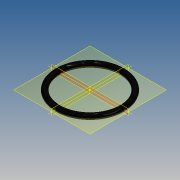
# Autodesk Inventor part: P030_OringCam
Saved by Autodesk Inventor 2021.3 (Build 253353000, 353)
## iProperties
Created: 2021-11-19
Part Number: P030_OringCam
Material: Générique
Document SubType Name: Modeling
Designer: gabri
Density: 1 g/cm^3
Appearance: Black
Author: gabri
Autodesk Inventor part; units mm, degrees
sketch "Sketch2" plane through (0, 0, 0) normal (0, 0, 1) x (1, 0, 0)
  circle A0 centre (0, 0) radius 17.75
  dimension "d0" = 35.5
  constraints: 1 centre point, 1 coincident
  measures "d0" diameter of A0
sketch "Sketch3" plane through (0, 0, 0) normal (0, 1, 0) x (-1, 0, 0)
  circle A0 centre (17.75, 0) radius 1.5
  line L0 (23.1, 0) -> (-3.85, 0) construction
  line L1 (0, -2.1) -> (0, 2.1) construction
  point P0 (0, 0)
  dimension "d1" = 3
  dimension "d2" = 17.75
  constraints: 1 centre point, 1 point on line
  measures "d1" diameter of A0
  measures "d2" distance from line of L1 A0.centre
sweep "Sweep1" add profiles "Sketch3" path "Sketch2"
body "Solid1"
